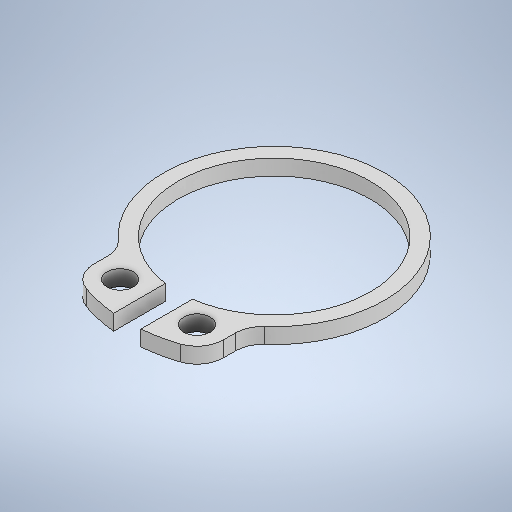
# Autodesk Inventor part: 49-01-004
Saved by Autodesk Inventor 2025.2 (Build 292293000, 293)
## iProperties
Created: 2024-11-28
Part Number: 49-01-004
Material: Generic
Document SubType Name: Modeling
Designer: Zvonko.Gabric
Density: 1 g/cm^3
Appearance: Default
Author: Zvonko.Gabric
Autodesk Inventor part; units mm, degrees
ref_plane "YZ Plane" through (0, 0, 0) normal (1, 0, 0) x (0, 1, 0)
ref_plane "XZ Plane" through (0, 0, 0) normal (0, 1, 0) x (-1, 0, 0)
ref_plane "XY Plane" through (0, 0, 0) normal (0, 0, 1) x (1, 0, 0)
sketch "Sketch1" plane through (0, 0, 0) normal (0, 1, 0) x (-1, 0, 0)
  line L0 (4.788, -33.3618) -> (4.788, -36.6836)
  line L1 (8.1671, -36.2479) -> (8.1671, -35.4556)
  line L2 (-0.2231, -35.4067) -> (-0.2231, -36.199)
  line L3 (3.0381, -36.6804) -> (3.0381, -33.3586)
  circle A0 centre (6.4671, -35.4556) radius 0.85
  circle A1 centre (1.4769, -35.4067) radius 0.85
  arc A2 (3.0381, -36.6804) -> (4.788, -36.6836) centre (3.9019, -42.7951) ccw
  arc A3 (7.028, -33.8508) -> (4.788, -33.3618) centre (3.9019, -42.7951) ccw
  arc A4 (8.1671, -35.4556) -> (7.028, -33.8508) centre (6.4671, -35.4556) ccw
  arc A5 (8.1671, -36.2479) -> (8.6017, -37.4732) centre (9.8649, -36.3356) ccw
  arc A6 (-0.7978, -37.4732) -> (8.6017, -37.4732) centre (3.9019, -42.7951) ccw
  arc A7 (-0.7978, -37.4732) -> (-0.2231, -36.199) centre (-1.9231, -36.199) ccw
  arc A8 (0.9161, -33.8019) -> (-0.2231, -35.4067) centre (1.4769, -35.4067) ccw
  arc A9 (3.0381, -33.3586) -> (0.9161, -33.8019) centre (3.9019, -42.7951) ccw
  point P0 (0, 0)
  dimension "d0" = 0
  dimension "d1" = 0
  dimension "d2" = 0
  dimension "d3" = 0
  dimension "d4" = 6.1754
  dimension "d5" = 7.1
  dimension "d6" = 1.7
  dimension "d7" = 1.7
  dimension "d8" = 1.7
  dimension "d9" = 1.7
  dimension "d10" = 1.7
  dimension "d11" = 1.7
  dimension "d12" = 9.476
  dimension "d13" = 9.4748
  dimension "d14" = 1.7499
  constraints: 16 point on circle, 10 centre point, 8 end point
  measures "d0" distance of A2.centre A6.centre
  measures "d1" distance of A1.centre A8.centre
  measures "d2" distance of A8.centre A1.centre
  measures "d3" distance of A0.centre A4.centre
  measures "d4" radius of A2
  measures "d5" radius of A6
  measures "d6" diameter of A0
  measures "d7" diameter of A1
  measures "d8" radius of A7
  measures "d9" radius of A5
  measures "d10" radius of A4
  measures "d11" radius of A8
  measures "d12" radius of A9
  measures "d13" radius of A3
  measures "d14" distance between parallel lines of L3 L0
extrude "Extrusion1" add sketch "Sketch1" along normal blind 1
body "Solid1"
